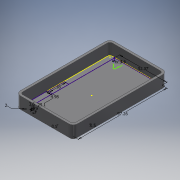
# Autodesk Inventor part: Case_3_inferior
Saved by Autodesk Inventor 2019 (Build 230136000, 136)
## iProperties
Created: 2018-11-27
Part Number: Case_3_inferior
Material: Steel, Mild, Welded
Document SubType Name: Modeling
Designer: cadcae
Density: 7.85 g/cm^3
Appearance: Smooth - Medium Gray
Author: cadcae
Autodesk Inventor part; units mm, degrees
ref_plane "YZ Plane" through (0, 0, 0) normal (1, 0, 0) x (0, 1, 0)
ref_plane "XZ Plane" through (0, 0, 0) normal (0, 1, 0) x (-1, 0, 0)
ref_plane "XY Plane" through (0, 0, 0) normal (0, 0, 1) x (1, 0, 0)
sketch "Sketch1" plane through (0, 0, 0) normal (0, 1, 0) x (-1, 0, 0)
  line L0 (-28.525, 48.63) -> (28.525, 48.63)
  line L1 (28.525, 48.63) -> (28.525, -48.63)
  line L2 (28.525, -48.63) -> (-28.525, -48.63)
  line L3 (-28.525, -48.63) -> (-28.525, 48.63)
  line L4 (-28.525, 48.63) -> (28.525, -48.63) construction
  line L5 (28.525, 48.63) -> (-28.525, -48.63) construction
  line L6 (29.025, -49.13) -> (29.025, 49.13)
  line L7 (29.025, 49.13) -> (-29.025, 49.13)
  line L8 (-29.025, 49.13) -> (-29.025, -49.13)
  line L9 (-29.025, -49.13) -> (29.025, -49.13)
  line L10 (31.425, 51.53) -> (31.425, -51.53)
  line L11 (31.425, -51.53) -> (-31.425, -51.53)
  line L12 (-31.425, -51.53) -> (-31.425, 51.53)
  line L13 (-31.425, 51.53) -> (31.425, 51.53)
  point P0 (0, 0)
  dimension "d0" = 97.26
  dimension "d1" = 57.05
  dimension "d2" = 0.5
  dimension "d3" = 2.4
  constraints: 28 end point, 6 parallel, 3 perpendicular, 2 midpoint, 1 horizontal, 6 other
  measures "d0" distance of L0.end L1.end
  measures "d1" distance of L1.end L2.end
  measures "d2" distance between parallel lines of L1 L6
  measures "d3" distance between parallel lines of L6 L10
extrude "Extrusion1" add sketch "Sketch1" against normal blind 14.87 contours L0 L1 L2 L3 | L9 L8 L7 L6 | L10 L11 L12 L13
fillet "Fillet2" radius 5 4 edges at (-31.425, -7.435, -51.53) (-31.425, -7.435, 51.53) (31.425, -7.435, 51.53) (31.425, -7.435, -51.53)
shell "Shell1" thickness 2.4 removed faces 1 at (10.475, 0, 15.51)
chamfer "Chamfer1" distance 2 angle 45 4 edges at (31.425, -14.87, 0) (0, -14.87, 51.53) (-31.425, -14.87, 0) (0, -14.87, -51.53)
sketch "Sketch7" plane through (-26.425, -12.47, -49.13) normal (0, 1, 0) x (1, 0, 0)
  arc A0 (55.45, -2.6) -> (52.85, 0) centre (52.85, -2.6) ccw projected
  line L0 (0, 0) -> (52.85, 0) projected
  arc A1 (0, 0) -> (-2.6, -2.6) centre (0, -2.6) ccw projected
  line L1 (-2.6, -95.66) -> (-2.6, -2.6) projected
  arc A2 (-2.6, -95.66) -> (0, -98.26) centre (0, -95.66) ccw projected
  line L2 (52.85, -98.26) -> (0, -98.26) projected
  arc A3 (52.85, -98.26) -> (55.45, -95.66) centre (52.85, -95.66) ccw projected
  line L3 (55.45, -2.6) -> (55.45, -95.66) projected
  line L4 (4.88, -97.76) -> (52.95, -97.76)
  line L5 (54.95, -95.76) -> (54.95, -2.5)
  line L6 (52.95, -0.5) -> (4.88, -0.5)
  line L7 (2.88, -2.5) -> (2.88, -95.76)
  arc A4 (2.88, -95.76) -> (4.88, -97.76) centre (4.88, -95.76) ccw
  arc A5 (4.88, -0.5) -> (2.88, -2.5) centre (4.88, -2.5) ccw
  arc A6 (54.95, -2.5) -> (52.95, -0.5) centre (52.95, -2.5) ccw
  arc A7 (52.95, -97.76) -> (54.95, -95.76) centre (52.95, -95.76) ccw
  line L8 (2.88, -68.66) -> (-2.1, -68.66)
  line L9 (-2.1, -68.66) -> (-2.1, -50.66)
  line L10 (-2.1, -50.66) -> (2.88, -50.66)
  line L11 (-2.1, -68.66) -> (-2.6, -68.66)
  circle A8 centre (5.88, -94.76) radius 1.8 construction
  line L12 (2.88, -89.96) -> (5.88, -89.96)
  arc A9 (10.68, -94.76) -> (5.88, -89.96) centre (5.88, -94.76) ccw
  line L13 (10.68, -94.76) -> (10.68, -98.26)
  line L14 (10.68, -98.26) -> (0, -98.26)
  line L15 (-2.6, -95.66) -> (-2.6, -68.66)
  arc A10 (-2.6, -95.66) -> (0, -98.26) centre (0, -95.66) ccw
  circle A11 centre (5.88, -3.5) radius 1.8 construction
  line L16 (14.2122, -3.7855) -> (13.3266, -11.4017)
  arc A12 (9.8285, -8.0807) -> (13.3266, -11.4017) centre (13.7908, -7.4099) ccw
  line L17 (9.8285, -8.0807) -> (7.2403, -6.8344)
  point P0 (26.425, -49.13)
  point P1 (54.95, -0.5)
  point P2 (54.95, -97.76)
  point P3 (2.88, -0.5)
  dimension "d43" = 52.07
  dimension "d44" = 97.26
  dimension "d45" = 0.5
  dimension "d46" = 0.5
  dimension "d47" = 2
  dimension "d48" = 18
  dimension "d49" = 4.98
  dimension "d50" = 29.1
  dimension "d51" = 3.6
  dimension "d52" = 3
  dimension "d53" = 3
  dimension "d54" = 3
  dimension "d55" = 3.6
  dimension "d56" = 3
  constraints: 28 end point, 14 point on circle, 12 point on line, 11 tangent, 9 centre point, 4 horizontal, 3 equal radius, 2 collinear, 2 parallel, 2 perpendicular, 2 vertical, 1 coincident, 1 concentric, 1 vertical alignment
  measures "d43" distance of point (2.88, -0.5) point (54.95, -0.5)
  measures "d44" distance of point (54.95, -0.5) point (54.95, -97.76)
  measures "d45" distance between parallel lines of L3 L5
  measures "d46" distance between parallel lines of L2 L4
  measures "d47" radius of A4
  measures "d48" distance of L8.end L9.end
  measures "d49" distance of L8.start L8.end
  measures "d50" distance between parallel lines of L4 L8
  measures "d51" diameter of A8
  measures "d52" distance from line of A8.centre L4
  measures "d53" distance from line of L7 A8.centre
  measures "d54" radial gap between concentric circles of A9 A8
  measures "d55" diameter of A11
  measures "d56" distance from line of L6 A11.centre
equation "\"d56\" = d52"
body "Solid1"
